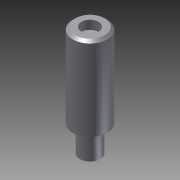
# Autodesk Inventor part: M211L01W-actuator
Saved by Autodesk Inventor 2011 SP1 (Build 150282100, 282)
## iProperties
Created: 2013-12-24
Part Number: M211L01W-actuator
Catalog Web Link: www.cadenas.de
Description: Series M2100 - LED Tipped Actuators -actuator-
Vendor: NKKSWITCHES
Document SubType Name: Modeling
Designer: PARTuser1
Manufacturer: NKKSWITCHES
Density: 1 g/cm^3
Category: PARTsolutions
Company: NKKSWITCHES
Title: M211L01W-actuator
Author: Cadenas PARTsolutions
PSOL_IDENT_0: {$CADENAS_DATA\23d-libs\nkkswitches\toggle\m2100\parts\m2100_actuator.prj},232 {VTYP=3D},{NB=M211L01
PSOL_IDENT_1: W-actuator},{LINA=M211L01W-actuator},{NN=Series M2100 - LED Tipped Actuators -actuator},{DATE=23.04.
PSOL_IDENT_2: 2009 12:56:26},{GEOMDATE=23.04.2009 12:14:00},{VERSION=},{LINEID=10},{LINESUBID=-1},{WBVAR=PLS,LCAT,
PSOL_IDENT_3: TMT,CMRT}  {NB=M211L01W-actuator},{LINA=M211L01W-actuator},{KT=DUMMY},{PN=M211L01W},{SRS=M21},{PLS=1
PSOL_IDENT_4: },{LCAT=L},{LCAT1= 'L','L - Isolated (Toggle)','T','T - Synchronous (Toggle)','R','R - Isolated (Roc
PSOL_IDENT_5: ker)','N','N - Synchronous (Rocker)','P','P - Isolated (Paddle)','J','J - Synchronous (Paddle)' },{A
PSOL_IDENT_6: CTUCLR=0.75,0.75,0.75,0.00},{TMT=01},{TMT1= '01','01 - Solder Lug with Threaded Bushing','02','02 -
PSOL_IDENT_7: Quick Connect with Threaded Bushing','03','03 - Straight PC with Threaded Bushing' },{CMRT=W}
CNS_NN: Series M2100 - LED Tipped Actuators -actuator
CNS_NB: M211L01W-actuator
CNS_NBSYN: $PN.-actuator
CNS_LINA: M211L01W-actuator
CNS_PN: M211L01W
CNS_SRS: M21
CNS_PLS: 1 - SPDT
CNS_LCAT: L - Isolated (Toggle)
CNS_LCAT1: 'L','L - Isolated (Toggle)','T','T - Synchronous (Toggle)','R','R - Isolated (Rocker)','N','N - Synchronous (Rocker)','P','P - Isolated (Paddle)','J','J - Synchronous (Paddle)'
CNS_ACTUCLR: 0.75,0.75,0.75,0.00
CNS_TMT: 01 - Solder Lug with Threaded Bushing
CNS_TMT1: '01','01 - Solder Lug with Threaded Bushing','02','02 - Quick Connect with Threaded Bushing','03','03 - Straight PC with Threaded Bushing'
CNS_CMRT: W - Silver; Rated 6A @ 125V AC
SUPPLIER: NKKSWITCHES
ARTICLENO: M211L01W-actuator
BOMINFO: M211L01W-actuator
CREATOR: CADENAS GmbH
Autodesk Inventor part; units mm, degrees
sketch "Sketch_1" plane through (0, 0, 0) normal (1, 0, 0) x (0, 1, 0)
  line L0 (-1.27, 0) -> (13.4366, 0)
  line L1 (13.4366, 0) -> (13.4366, -1.2446)
  line L2 (13.4366, -1.2446) -> (14.7066, -1.2446)
  line L3 (14.7066, -1.2446) -> (14.7066, -2.1427)
  line L4 (14.7066, -2.1427) -> (14.3474, -2.5019)
  line L5 (14.3474, -2.5019) -> (2.54, -2.5019)
  line L6 (2.54, -2.5019) -> (2.54, -1.4859)
  line L7 (2.54, -1.4859) -> (-1.27, -1.4859)
  line L8 (-1.27, -1.4859) -> (-1.27, 0)
  line L9 (-1.27, 0) -> (13.4366, 0)
  constraints: 20 end point
revolve "Revolution1" add sketch "Sketch_1" angle 360 about axis through (0, -1.27, 0) along (0, -1, 0)
ref_plane "paddle_to_bracket_XY" through (0, -1.3716, 0) normal (0, 0, -1) x (1, 0, 0)
ref_plane "paddle_to_bracket_YZ" through (0, -1.3716, 0) normal (1, 0, 0) x (0, -1, 0)
ref_plane "paddle_to_bracket_ZX" through (0, -1.3716, 0) normal (0, -1, 0) x (0, 0, -1)
ref_plane "paddle_to_led_XY" through (0, 13.8525, 0) normal (0, 1, 0) x (1, 0, 0)
ref_plane "paddle_to_led_YZ" through (0, 13.8525, 0) normal (1, 0, 0) x (0, 0, -1)
ref_plane "paddle_to_led_ZX" through (0, 13.8525, 0) normal (0, 0, -1) x (0, 1, 0)
ref_plane "paddle_to_led_green_XY" through (0, 13.8525, 0) normal (0, 1, 0) x (1, 0, 0)
ref_plane "paddle_to_led_green_YZ" through (0, 13.8525, 0) normal (1, 0, 0) x (0, 0, -1)
ref_plane "paddle_to_led_green_ZX" through (0, 13.8525, 0) normal (0, 0, -1) x (0, 1, 0)
ref_plane "rocker_to_bracket_XY" through (0, 1.778, 0) normal (0, -1, 0) x (1, 0, 0)
ref_plane "rocker_to_bracket_YZ" through (0, 1.778, 0) normal (1, 0, 0) x (0, 0, 1)
ref_plane "rocker_to_bracket_ZX" through (0, 1.778, 0) normal (0, 0, 1) x (0, -1, 0)
ref_plane "toggle_to_bc_XY" through (0, 0, 0) normal (0, 1, 0) x (1, 0, 0)
ref_plane "toggle_to_bc_YZ" through (0, 0, 0) normal (1, 0, 0) x (0, 0, -1)
ref_plane "toggle_to_bc_ZX" through (0, 0, 0) normal (0, 0, -1) x (0, 1, 0)
ref_plane "toggle_to_led_XY" through (0, 13.4366, 0) normal (0, 1, 0) x (1, 0, 0)
ref_plane "toggle_to_led_YZ" through (0, 13.4366, 0) normal (1, 0, 0) x (0, 0, -1)
ref_plane "toggle_to_led_ZX" through (0, 13.4366, 0) normal (0, 0, -1) x (0, 1, 0)
ref_plane "toggle_to_led_green_XY" through (0, 13.4366, 0) normal (0, 1, 0) x (1, 0, 0)
ref_plane "toggle_to_led_green_YZ" through (0, 13.4366, 0) normal (1, 0, 0) x (0, 0, -1)
ref_plane "toggle_to_led_green_ZX" through (0, 13.4366, 0) normal (0, 0, -1) x (0, 1, 0)
body "Solid1"
